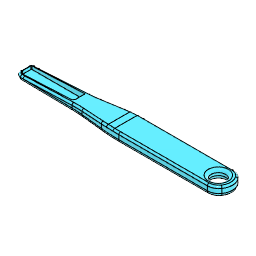
Nozzle_brush A5 (Autodesk Fusion 360 design; units mm, degrees)
Autodesk Fusion 360 part; units mm, degrees
sketch "Sketch1" plane through (0, 0, 0) normal (0, 0, 1) x (1, 0, 0)
  arc A0 (-18.55, -2.05) -> (-16.55, -4.05) centre (-16.55, -2.05) ccw
  line L0 (-16.55, -4.05) -> (16.55, -4.05)
  arc A1 (16.55, -4.05) -> (18.55, -2.05) centre (16.55, -2.05) ccw
  line L1 (18.55, -2.05) -> (18.55, 4.05)
  line L2 (18.55, 4.05) -> (-18.55, 4.05)
  line L3 (-18.55, 4.05) -> (-18.55, -2.05)
  line L4 (-19.95, 5.65) -> (48.55, 6.7)
  line L5 (48.55, 6.7) -> (48.55, -6.7)
  line L6 (48.55, -6.7) -> (-19.95, -5.65)
  line L7 (-19.95, -5.65) -> (-19.95, 5.65)
  line L8 (48.55, 9) -> (118.55, 9)
  line L9 (118.55, 9) -> (118.55, -9)
  line L10 (118.55, -9) -> (48.55, -9)
  line L11 (48.55, -9) -> (48.55, 9)
  line L12 (48.55, 9) -> (23.55, 6.3168)
  line L13 (48.55, -9) -> (23.55, -6.3168)
  arc A2 (118.55, -9) -> (118.55, 9) centre (114.8, 0) ccw
  circle A3 centre (114.8, 0) radius 5
  point P0 (48.55, 0)
  point P1 (48.55, 0)
  point P2 (124.55, 0)
  point P3 (18.55, 6.2401)
  dimension "d1" = 1.4
  dimension "d3" = 30
  dimension "d5" = 18
  dimension "d6" = 70
  dimension "d7" = 5
  dimension "d8" = 6
  dimension "d33" = 10
  dimension "d78" = 1.6
  dimension "d79" = 1.6
  dimension "d80" = 13.4
  dimension "d82" = 2.1901
  constraint vertical L5
  constraint vertical L7
  constraint horizontal L8
  constraint vertical L9
  constraint horizontal L10
  constraint vertical L11
  constraint midpoint L5 P1
  constraint midpoint L11 P1
  constraint coincident P1 P0
  constraint coincident L4 L12.end
  constraint coincident L6 L13.end
  constraint vertical L12.end L13.end
  constraint midpoint A2 P2
  constraint concentric A2 A3
  constraint vertical L1.end P3
  constraint coincident L4 P3
  constraint horizontal origin P1
  measures "d1" distance of L3 L7
  measures "d3" distance of L1 L11
  measures "d5" distance of L8.end L9.end
  measures "d6" distance of L8.start L8.end
  measures "d7" horizontal distance of L1.end L12.end
  measures "d8" distance of L9 P2
  measures "d33" diameter of A3
  measures "d78" vertical distance of L2.end L4.start
  measures "d79" vertical distance of A0.end L6.end
  measures "d80" distance of L4.end L5.end
  measures "d82" distance of L1.end P3
extrude "Extrude1" add sketch "Sketch1" along normal blind 3 contours A0 L0 A1 L1 L2 L3 | L4 L5 L6 L7 L11 | L4 L11 L12 | L5 L8 L9 L10 L11 A3 | L6 L11 L13 | L9 A2 A3
extrude "Extrude2" cut sketch "Sketch1" against normal blind 2.2 from surface at 3 contours A0 L0 A1 L1 L2 L3
extrude "Extrude3" add sketch "Sketch1" along normal blind 6 contours L5 L8 L9 L10 L11 A3 | L9 A2 A3
extrude "Extrude4" add 1 faces at (40.2167, -2.1056, 3) along direction (0, 0, 1) up to surface (3 mm away)
sketch "Sketch2" plane through (0, 4.05, 0) normal (0, -1, 0) x (1, 0, 0)
  line L0 (-14.55, 3) -> (48.5717, 6.001)
  line L1 (48.55, 6) -> (48.5717, 6.001)
  line L2 (-14.55, 3) -> (-19.95, 3)
  line L3 (-19.95, 0) -> (23.55, 0)
  line L4 (23.55, 0) -> (23.55, 6)
  line L5 (23.55, 6) -> (-19.95, 6)
  line L6 (-19.95, 6) -> (-19.95, 0)
  line L7 (23.55, 0) -> (48.55, 0)
  line L8 (48.55, 0) -> (48.55, 6)
  line L9 (48.55, 6) -> (23.55, 6)
  line L10 (23.55, 6) -> (23.55, 0)
  line L11 (48.55, 0) -> (118.55, 0)
  line L12 (118.55, 0) -> (118.55, 6)
  line L13 (118.55, 6) -> (48.55, 6)
  line L14 (48.55, 6) -> (48.55, 0)
  line L15 (-18.55, 6) -> (-18.55, 0.8)
  line L16 (-18.55, 0.8) -> (18.55, 0.8)
  line L17 (18.55, 0.8) -> (18.55, 6)
  line L18 (18.55, 6) -> (-18.55, 6)
  dimension "d83" = 3
  dimension "d84" = 70
  dimension "d85" = 4
  constraint collinear L0 L1
  constraint horizontal L2
  constraint coincident L2.end L6
  constraint coincident L1.start L13
  measures "d83" distance of L2 L3
  measures "d84" distance of L1.start L12.end
  measures "d85" distance of L0.start L15
extrude "Extrude5" cut sketch "Sketch2" along normal mid plane 100 contours L0 L4 L9 L10 | L0 L4 L5 L10 L17 | L0 L2 L5 L15 L17 L18 | L2 L5 L6 L15
fillet "Fillet11" radius 80 2 edges at (23.55, -6.3168, 2.4057) (23.55, 6.3168, 2.4057)
fillet "Fillet12" radius 120 2 edges at (48.55, 9, 3) (48.55, -9, 3)
fillet "Fillet16" radius 3.6 1 edges at (-19.95, -5.65, 1.5)
fillet "Fillet17" radius 2 1 edges at (-19.95, 5.65, 1.5)
fillet "Fillet5" radius 8 2 edges at (118.55, -9, 1.5) (118.55, 9, 1.5)
fillet "Fillet14" radius 100 1 edges at (48.55, 0, 6)
fillet "Fillet18" radius 0.4 2 edges at (-18.55, 4.05, 1.9) (18.55, 4.05, 2.6868)
fillet "Fillet7" radius 1.2 22 edges at (85.6037, -9, 6) (119.9394, -8.0912, 6) (124.55, 0, 6) (119.9394, 8.0912, 6) (85.6037, 9, 6) (52.9483, 8.9829, 6) (48.5607, 8.8286, 5.972) (44.1696, 8.5129, 5.7917) (34.6804, 7.5114, 5.3406) (23.5449, 6.4006, 4.8112) (2.6671, 5.9967, 3.8186) (52.9483, -8.9829, 6) (48.5607, -8.8286, 5.972) (44.1696, -8.5129, 5.7917) (34.6804, -7.5114, 5.3406) (23.5449, -6.4006, 4.8112) (2.6671, -5.9967, 3.8186) (-19.95, 0.7878, 3) (-19.375, 5.0838, 3) (-16.2653, 5.7065, 3) (-18.915, -4.6308, 3) (-15.4776, -5.7186, 3)
chamfer "Chamfer1" distance 0.8 angle 45 16 edges at (85.6037, -9, 0) (48.5592, -8.8286, 0) (34.6804, -7.5114, 0) (23.5449, -6.4006, 0) (1.7395, -5.9825, 0) (-18.915, -4.6308, 0) (-19.95, 0.7878, 0) (-19.375, 5.0838, 0) (0.9518, 5.9704, 0) (23.5449, 6.4006, 0) (34.6804, 7.5114, 0) (48.5592, 8.8286, 0) (85.6037, 9, 0) (119.9394, 8.0912, 0) (124.55, 0, 0) (119.9394, -8.0912, 0) measured on face at (73.2475, 0, 0) measured on face at (49.2704, -8.8645, 3.1642) measured on face at (73.2475, 0, 0) measured on face at (21.9467, -6.3188, 2.3513) measured on face at (73.2475, 0, 0) measured on face at (-19.946, -2.2744, 1.2) measured on face at (73.2475, 0, 0) measured on face at (-19.9478, 3.7747, 0.6) measured on face at (73.2475, 0, 0) measured on face at (21.9467, 6.3188, 2.3513) measured on face at (37.1941, 7.7812, 2.7644) measured on face at (49.2704, 8.8645, 3.1642) measured on face at (73.2475, 0, 0) measured on face at (122.3553, 6.1532, 3.2) measured on face at (123.2703, -4.8288, 1.6) measured on face at (116.6027, -8.9916, 3.2)
fillet "Fillet13" radius 2.4 16 edges at (124.55, 0, 0.8) (119.9394, -8.0912, 0.8) (85.6037, -9, 0.8) (48.5592, -8.8286, 0.8) (34.6804, -7.5114, 0.8) (23.5449, -6.4006, 0.8) (1.7395, -5.9825, 0.8) (-18.915, -4.6308, 0.8) (-19.95, 0.7878, 0.8) (-19.375, 5.0838, 0.8) (0.9518, 5.9704, 0.8) (23.5449, 6.4006, 0.8) (34.6804, 7.5114, 0.8) (48.5592, 8.8286, 0.8) (85.6037, 9, 0.8) (119.9394, 8.0912, 0.8)
chamfer "Chamfer3" distance 1 angle 45 1 edges at (110.1384, 1.8081, 0)
fillet "Fillet9" radius 3 1 edges at (110.1384, -1.8081, 1)
fillet "Fillet15" radius 2 1 edges at (110.1384, 1.8081, 6)
equation "d10 = head_tip_thick"
equation "d13 = -( head_tip_thick - back_of_bristles_thick )"
equation "d39 = body_thick"
equation "d79 = d78"
equation "d83 = head_tip_thick"
equation "head_tip_thick = 3 mm"
equation "body_thick = 6 mm"
equation "back_of_bristles_thick = 0.8 mm"
